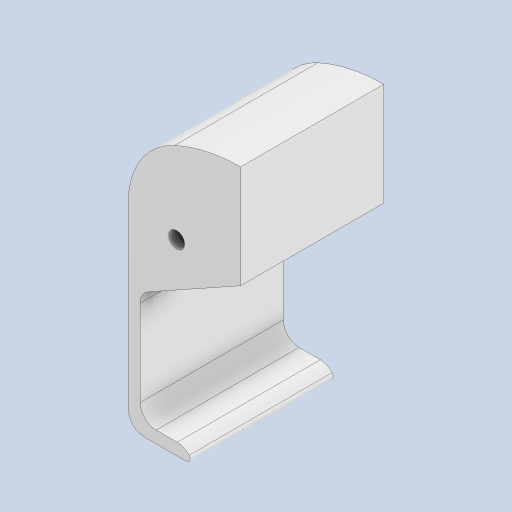
# Autodesk Inventor part: Gancio1
Saved by Autodesk Inventor 2023.2 (Build 272271030, 271C)
## iProperties
Created: 2023-02-08
Part Number: Gancio1
Material: Plastica ABS
Document SubType Name: Modeling
Designer: daler
Density: 1.06 g/cm^3
Appearance: Liscia - Bianco
Mass: 7.54125 g
Surface Area: 30.3226 cm^2
Volume: 7.11439 cm^3
Author: daler
Autodesk Inventor part; units mm, degrees
ref_plane "YZ Plane" through (0, 0, 0) normal (1, 0, 0) x (0, 1, 0)
ref_plane "XZ Plane" through (0, 0, 0) normal (0, 1, 0) x (-1, 0, 0)
ref_plane "XY Plane" through (0, 0, 0) normal (0, 0, 1) x (1, 0, 0)
sketch "Schizzo1" plane through (0, 0, 0) normal (0, 0, 1) x (1, 0, 0)
  line L0 (9.6257, 10.2674) -> (9.6257, -2.6852)
  arc A0 (9.6257, 10.2674) -> (-4.5165, 4.4095) centre (9.6257, -9.7326) ccw
  line L1 (-0.3743, -9.7326) -> (-4.5165, 4.4095) construction
  line L2 (9.6257, 0.2674) -> (-4.5165, 4.4095) construction
  line L3 (4.6257, -4.7326) -> (9.6257, 0.2674) construction
  line L4 (-4.5165, 4.4095) -> (4.6257, -4.7326) construction
  line L5 (9.6257, 0.2674) -> (-2.4454, -2.6616) construction
  circle A1 centre (1.5783, -1.6852) radius 1
  line L6 (-4.5165, 4.4095) -> (-4.5165, -25.2326)
  line L7 (-4.5165, -25.2326) -> (-3.0165, -25.2326)
  line L8 (-3.0165, -23.7326) -> (-3.0165, -9.7326)
  line L9 (-3.0165, -25.2326) -> (3.5901, -25.2326)
  line L10 (3.5901, -25.2326) -> (3.5901, -23.7326)
  line L11 (3.5901, -23.7326) -> (-3.0165, -23.7326)
  line L12 (-3.0165, -9.7326) -> (9.6257, -2.6852)
  point P0 (0, 0)
  dimension "d6" = 2
  dimension "d24" = 1.5
  dimension "d27" = 14
  dimension "d28" = 1.5
  constraints: 26 end point, 3 point on line, 2 centre point, 2 horizontal, 2 perpendicular, 2 point on circle, 1 midpoint, 1 vertical
  measures "d6" diameter of A1
  measures "d24" distance between parallel lines of L6 L8
  measures "d27" distance of L8.start L8.end
  measures "d28" distance between parallel lines of L9 L11
extrude "Estrusione1" add sketch "Schizzo1" along normal blind 18
fillet "Raccordo11" radius 2 4 edges at (-3.0165, -9.7326, 9) (-3.0165, -23.7326, 9) (-4.5165, -25.2326, 9) (3.5901, -23.7326, 9)
fillet "Raccordo12" radius 10 1 edges at (-4.5165, 4.4095, 9)
fillet "Raccordo13" radius 0.5 1 edges at (3.5901, -25.2326, 9)
